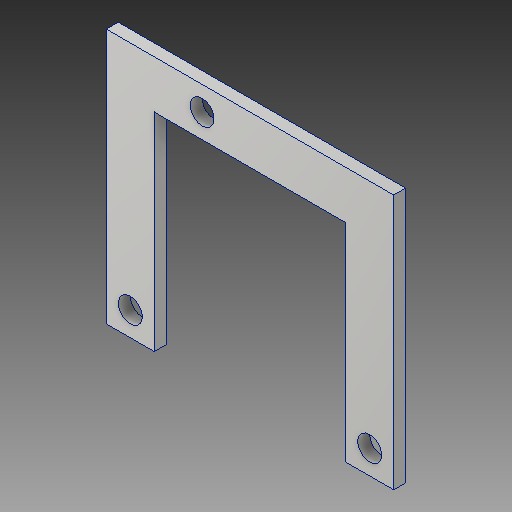
# Autodesk Inventor part: bogie_square_alt
Saved by Autodesk Inventor 2018.1 (Build 221171000, 171)
## iProperties
Created: 2017-10-26
Part Number: bogie_square_alt
Material: アルミニウム 6061
Document SubType Name: Modeling
Designer: Kakeru Yamashita
Density: 2.7 g/cm^3
Appearance: アルミニウム - フラット
Mass: 75.9831 g
Surface Area: 148.6 cm^2
Volume: 28.1419 cm^3
Author: Kakeru Yamashita
Autodesk Inventor part; units mm, degrees
ref_plane "YZ Plane" through (0, 0, 0) normal (1, 0, 0) x (0, 1, 0)
ref_plane "XZ Plane" through (0, 0, 0) normal (0, 1, 0) x (-1, 0, 0)
ref_plane "XY Plane" through (0, 0, 0) normal (0, 0, 1) x (1, 0, 0)
sketch "スケッチ1" plane through (0, 0, 0) normal (0, 1, 0) x (-1, 0, 0)
  line L0 (127.92, 0) -> (-21.32, 0) projected
  line L1 (0, -84) -> (0, 84) projected
  line L2 (106.6, 0) -> (106.6, -60)
  line L3 (106.6, -60) -> (0, -60)
  line L4 (0, -40) -> (86.6, -40)
  line L5 (86.6, -40) -> (86.6, 0)
  line L6 (106.6, 0) -> (106.6, 60)
  line L7 (106.6, 60) -> (0, 60)
  line L8 (0, 40) -> (86.6, 40)
  line L9 (86.6, 40) -> (86.6, 0)
  line L10 (0, 60) -> (0, 40)
  line L11 (0, -40) -> (0, -60)
  point P0 (0, 0)
  dimension "d0" = 20
  dimension "d4" = 20
  dimension "d15" = 60
  dimension "d16" = 106.6
  constraints: 20 end point, 4 point on line, 4 symmetric about line, 2 collinear, 2 perpendicular, 1 parallel
  measures "d0" distance between parallel lines of L5 L2
  measures "d4" distance between parallel lines of L3 L4
  measures "d15" distance between parallel lines of L0 L3
  measures "d16" distance between parallel lines of L1 L2
extrude "押し出し1" add sketch "スケッチ1" along normal blind 5 contours L2 L3 L1 L4 L5 L0 | L0 L9 L8 L1 L7 L6
sketch "スケッチ2" plane through (0, 5, 0) normal (0, 1, 0) x (1, 0, 0)
  circle A0 centre (-10, -50) radius 5
  line L0 (0, -60) -> (0, -40) projected
  line L1 (-106.6, -60) -> (0, -60) projected
  line L2 (-127.92, 0) -> (21.32, 0) projected
  circle A1 centre (-10, 50) radius 5
  circle A2 centre (-96.6, -20) radius 5
  line L3 (-86.6, -40) -> (-86.6, 40) projected
  point P0 (0, 0)
  dimension "d8" = 10
  dimension "d9" = 10
  dimension "d10" = 10
  dimension "d11" = 10
  dimension "d12" = 10
  dimension "d17" = 30
  constraints: 3 centre point, 1 symmetric about line, 1 other
  measures "d8" diameter of A0
  measures "d9" distance from line of L0 A0.centre
  measures "d10" distance from line of L1 A0.centre
  measures "d11" diameter of A2
  measures "d12" distance from line of L3 A2.centre
  measures "d17" vertical distance of A0.centre A2.centre
extrude "押し出し2" cut sketch "スケッチ2" against normal blind 5
